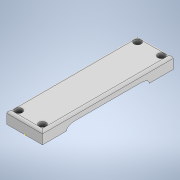
# Autodesk Inventor part: TestClosedLoopBearing
Saved by Autodesk Inventor 2022 (Build 260153000, 153)
## iProperties
Created: 2022-03-13
Part Number: TestClosedLoopBearing
Material: Generic
Document SubType Name: Modeling
Designer: Jorian Brusind
Density: 1 g/cm^3
Appearance: Default
Author: Jorian Brusind
Autodesk Inventor part; units mm, degrees
ref_plane "YZ Plane" through (0, 0, 0) normal (1, 0, 0) x (0, 1, 0)
ref_plane "XZ Plane" through (0, 0, 0) normal (0, 1, 0) x (-1, 0, 0)
ref_plane "XY Plane" through (0, 0, 0) normal (0, 0, 1) x (1, 0, 0)
sketch "Sketch1" plane through (0, 0, 0) normal (0, 1, 0) x (-1, 0, 0)
  line L0 (-13.75, -50) -> (13.75, -50)
  line L1 (13.75, -50) -> (13.75, 50)
  line L2 (13.75, 50) -> (-13.75, 50)
  line L3 (-13.75, 50) -> (-13.75, -50)
  line L4 (-13.75, -50) -> (13.75, 50) construction
  line L5 (13.75, -50) -> (-13.75, 50) construction
  line L6 (-13.75, 0) -> (-12.625, 0)
  line L7 (-12.625, -27.5) -> (-12.625, 27.5) construction
  line L8 (-8, -27.5) -> (-8, 27.5)
  line L9 (-17.25, 27.5) -> (-17.25, -27.5)
  arc A0 (-17.25, -27.5) -> (-8, -27.5) centre (-12.625, -27.5) ccw
  arc A1 (-8, 27.5) -> (-17.25, 27.5) centre (-12.625, 27.5) ccw
  line L10 (-12.625, 0) -> (42.375, 0) construction
  line L11 (-12.625, 27.5) -> (-3.375, 27.5)
  line L12 (-12.625, 0) -> (5.875, 0)
  line L13 (5.875, -27.5) -> (5.875, 27.5) construction
  line L14 (10.5, -27.5) -> (10.5, 27.5)
  line L15 (1.25, 27.5) -> (1.25, -27.5)
  arc A2 (1.25, -27.5) -> (10.5, -27.5) centre (5.875, -27.5) ccw
  arc A3 (10.5, 27.5) -> (1.25, 27.5) centre (5.875, 27.5) ccw
  line L16 (5.875, 0) -> (60.875, 0) construction
  arc A4 (5.875, 27.5) -> (-12.625, 27.5) centre (-3.375, 27.5) ccw construction
  arc A5 (10.5, 27.5) -> (-17.25, 27.5) centre (-3.375, 27.5) ccw
  arc A6 (1.25, 27.5) -> (-8, 27.5) centre (-3.375, 27.5) ccw
  arc A7 (1.25, 27.5) -> (10.5, 27.5) centre (5.875, 27.5) ccw
  arc A8 (-17.25, 27.5) -> (-8, 27.5) centre (-12.625, 27.5) ccw
  arc A9 (-12.625, -27.5) -> (5.875, -27.5) centre (-3.375, -27.5) ccw construction
  arc A10 (-17.25, -27.5) -> (10.5, -27.5) centre (-3.375, -27.5) ccw
  arc A11 (-8, -27.5) -> (1.25, -27.5) centre (-3.375, -27.5) ccw
  arc A12 (-8, -27.5) -> (-17.25, -27.5) centre (-12.625, -27.5) ccw
  arc A13 (10.5, -27.5) -> (1.25, -27.5) centre (5.875, -27.5) ccw
  line L17 (-12.625, 0) -> (-12.625, -27.5)
  line L18 (-12.625, 0) -> (-12.625, 27.5)
  line L19 (5.875, 27.5) -> (5.875, -27.5)
  arc A14 (-12.625, -27.5) -> (5.875, -27.5) centre (-3.375, -27.5) ccw
  arc A15 (5.875, 27.5) -> (-12.625, 27.5) centre (-3.375, 27.5) ccw
  line L20 (-13.75, 0) -> (-18, 0)
  line L21 (-12.625, 27.5) -> (-15.445, 27.5)
  point P0 (0, 0)
  dimension "d0" = 27.5
  dimension "d1" = 100
  dimension "d4" = 90
  dimension "d5" = 9.25
  dimension "d6" = 9.25
  dimension "d7" = 18.5
  dimension "d8" = 27.5
  dimension "d9" = 90
  dimension "d10" = 9.25
  dimension "d11" = 9.25
  dimension "d12" = 9.25
  dimension "d13" = 9.25
  dimension "d14" = 9.25
  dimension "d22" = 9.25
  dimension "d43" = 3.5
  dimension "d44" = 2.82
  dimension "d46" = 9.25
  constraints: 48 end point, 32 point on circle, 16 centre point, 16 tangent, 7 horizontal, 6 parallel, 5 midpoint, 5 perpendicular, 1 collinear, 1 point on line
  measures "d0" distance of L2.end L1.end
  measures "d1" distance of L1.end L0.end
  measures "d4" angle of L10 L7
  measures "d5" diameter of A1
  measures "d6" distance of L7.end L11.end
  measures "d7" distance of L6.end L12.end
  measures "d8" distance of L12.end L13.end
  measures "d9" angle of L16 L13
  measures "d10" diameter of A3
  measures "d11" radius of A4
  measures "d12" diameter of A7
  measures "d13" radius of A9
  measures "d14" diameter of A13
  measures "d22" radius of A14
  measures "d43" distance between parallel lines of L3 L9
  measures "d44" distance of L7.end L21.end
  measures "d46" radius of A15
sketch "Sketch2" plane through (0, 0, 0) normal (0, 1, 0) x (-1, 0, 0)
  line L0 (-15, -55) -> (15, -55)
  line L1 (15, -55) -> (15, 55)
  line L2 (15, 55) -> (-15, 55)
  line L3 (-15, 55) -> (-15, -55)
  line L4 (-15, -55) -> (15, 55) construction
  line L5 (15, -55) -> (-15, 55) construction
  point P0 (0, 0)
  dimension "d15" = 30
  dimension "d16" = 110
  constraints: 12 end point, 2 midpoint, 2 parallel, 1 horizontal, 1 perpendicular
  measures "d15" distance of L2.end L1.end
  measures "d16" distance of L1.end L0.end
extrude "Extrusion1" add sketch "Sketch2" along normal blind 10
ref_plane "Work Plane1" through (15, 0, -5) normal (0, 0, -1) x (-1, 0, 0)
sketch "Sketch3" plane through (15, 0, -5) normal (0, 0, -1) x (-1, 0, 0)
  line L0 (0, 0) -> (2.5, 0)
  circle A0 centre (2.5, 0) radius 4.625
  point P0 (15, 0)
  dimension "d20" = 2.5
  dimension "d21" = 9.25
  constraints: 2 end point, 1 centre point, 1 coincident, 1 horizontal
  measures "d20" distance of L0.start L0.end
  measures "d21" diameter of A0
sweep "Sweep1" cut profiles "Sketch3" path "Sketch1" path curves L18 A15 L19 A14 L17
sketch "Sketch4" plane through (0, 0, 0) normal (0, -1, 0) x (1, 0, 0)
  line L0 (-15, -55) -> (-15, 55) projected
  line L1 (-15, -55) -> (-15, -50)
  line L2 (-15, -50) -> (-10, -50)
  line L3 (-15, 55) -> (-15, 50)
  line L4 (-15, 50) -> (-10, 50)
  circle A0 centre (-10, -50) radius 3
  circle A1 centre (-10, 50) radius 3
  line L5 (15, -55) -> (15, -50)
  line L6 (15, -50) -> (10, -50)
  circle A2 centre (10, -50) radius 3
  line L7 (-15, 55) -> (15, 55) projected
  line L8 (15, 55) -> (15, 50)
  line L9 (15, 55) -> (15, -55) projected
  line L10 (15, 50) -> (10, 50)
  circle A3 centre (10, 50) radius 3
  point P0 (0, 0)
  dimension "d26" = 5
  dimension "d27" = 5
  dimension "d28" = 5
  dimension "d29" = 5
  dimension "d30" = 6
  dimension "d31" = 6
  dimension "d37" = 5
  dimension "d38" = 5
  dimension "d39" = 6
  dimension "d40" = 5
  dimension "d41" = 5
  dimension "d42" = 6
  constraints: 16 end point, 4 centre point, 4 coincident, 4 perpendicular, 3 point on line, 1 vertical
  measures "d26" distance of L0.start L1.end
  measures "d27" distance of L1.end L2.end
  measures "d28" distance of L0.end L3.end
  measures "d29" distance of L3.end L4.end
  measures "d30" diameter of A0
  measures "d31" diameter of A1
  measures "d37" distance of L5.start L5.end
  measures "d38" distance of L5.end L6.end
  measures "d39" diameter of A2
  measures "d40" distance of L7.end L8.end
  measures "d41" distance of L8.end L10.end
  measures "d42" diameter of A3
extrude "Extrusion2" cut sketch "Sketch4" against normal blind 10
fillet "Fillet1" radius 2 4 edges at (0, 10, -55) (-15, 10, 0) (15, 10, 0) (0, 10, 55)
fillet "Fillet3" radius 2 4 edges at (3.375, 0, 32) (-1.125, 0, 0) (3.375, 0, -32) (7.875, 0, 0)
sketch "Sketch5" plane through (-15, 0, 55) normal (0, 0, 1) x (1, 0, 0)
  point P0 (15, 0)
equation "\"d0\" = length"
equation "\"d5\" = radius"
equation "\"d6\" = radius"
equation "\"d7\" = 2 * radius"
equation "\"d10\" = radius"
equation "\"d11\" = radius"
equation "\"d12\" = radius"
equation "\"d13\" = radius"
equation "\"d14\" = radius"
equation "\"d22\" = radius"
equation "\"d46\" = radius"
equation "\"radius\" = 9.25"
equation "\"length\" = 27.5"
body "Solid1"
